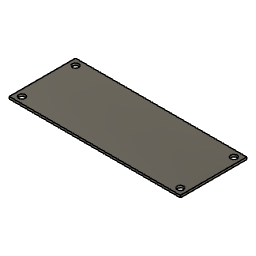
substrate3 (Autodesk Fusion 360 design; units mm, degrees)
Autodesk Fusion 360 part; units mm, degrees
sketch "スケッチ1" plane through (0, 0, 0) normal (0, 0, 1) x (1, 0, 0)
  line L0 (0, 0) -> (80, 0)
  line L1 (80, 0) -> (80, 31)
  line L2 (80, 31) -> (0, 31)
  line L3 (0, 31) -> (0, 0)
  line L4 (0, 31) -> (3, 31)
  line L5 (0, 28) -> (0, 31)
  circle A0 centre (3, 28) radius 1.5
  line L6 (0, 0) -> (3, 0)
  line L7 (0, 3) -> (0, 0)
  circle A1 centre (3, 3) radius 1.5
  line L8 (80, 0) -> (77, 0)
  line L9 (80, 3) -> (80, 0)
  line L10 (80, 31) -> (77, 31)
  line L11 (80, 28) -> (80, 31)
  circle A2 centre (77, 28) radius 1.5
  circle A3 centre (77, 3) radius 1.5
  dimension "d1" = 80
  dimension "d2" = 31
  dimension "d3" = 3
  dimension "d4" = 3
  dimension "d5" = 3
  dimension "d6" = 3
  dimension "d7" = 3
  dimension "d8" = 3
  dimension "d9" = 3
  constraint horizontal L0
  constraint vertical L1
  constraint horizontal L2
  constraint vertical L3
  constraint coincident L0.start L3.end
  constraint horizontal L4
  constraint vertical L5
  constraint horizontal L6
  constraint vertical L7
  constraint horizontal L8
  constraint vertical L9
  constraint horizontal L10
  constraint vertical L11
  measures "d1" distance of L0.start L0.end
  measures "d2" distance of L0.start L2.end
  measures "d3" distance of L2.end L4.end
  measures "d4" distance of L2.end L5.start
  measures "d5" diameter of A0
  measures "d6" distance of L0.start L6.end
  measures "d7" diameter of A1
  measures "d8" diameter of A2
  measures "d9" diameter of A3
extrude "押し出し1" add sketch "スケッチ1" along normal blind 1
